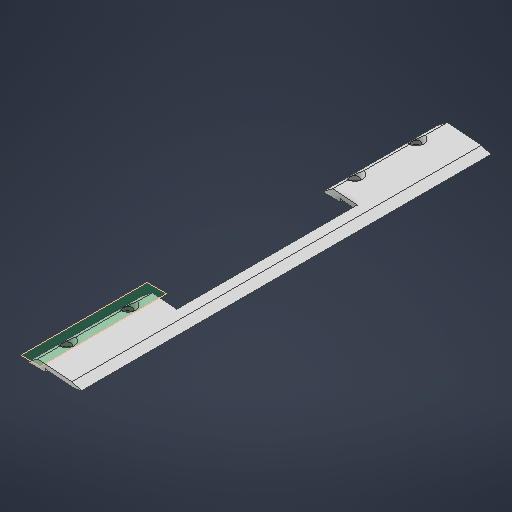
# Autodesk Inventor part: przódv3
Saved by Autodesk Inventor 2026.2 (Build 302298010, 298A)
## iProperties
Created: 2026-05-13
Part Number: przódv3
Material: Generic
Document SubType Name: Modeling
Designer: karol
Density: 1 g/cm^3
Appearance: Default
Author: karol
Autodesk Inventor part; units mm, degrees
ref_plane "YZ Plane" through (0, 0, 0) normal (1, 0, 0) x (0, 1, 0)
ref_plane "XZ Plane" through (0, 0, 0) normal (0, 1, 0) x (-1, 0, 0)
ref_plane "XY Plane" through (0, 0, 0) normal (0, 0, 1) x (1, 0, 0)
sketch "Sketch1" plane through (0, 0, 0) normal (0, 0, 1) x (1, 0, 0)
  line L0 (0.1259, -2.059) -> (22.8182, -5.8085) projected
  line L1 (22.8182, -5.8085) -> (24.1224, 2.0845) projected
  line L2 (11.2963, 4.2038) -> (24.1224, 2.0845) projected
  line L3 (11.2963, 4.2038) -> (0.6373, 1.036) projected
  line L4 (0.6373, 1.036) -> (0.1259, -2.059) projected
  line L5 (0, 0) -> (0, 2) projected
  line L6 (0, 2) -> (-6.5, 2) projected
  line L7 (-6.5, 0) -> (-6.5, 2) projected
  line L8 (0, 0) -> (-6.5, 0) projected
  line L9 (-6.5, 2) -> (0, 2)
  line L10 (-6.5, 2) -> (0, 2)
  line L11 (0, 2) -> (0, 3.5)
  line L12 (0, 3.5) -> (11.2963, 4.2038)
  line L13 (-2.7633, 4.8337) -> (11.2028, 5.7038)
  line L14 (11.2028, 5.7038) -> (11.2963, 4.2038)
  line L15 (-2.7633, 4.8337) -> (-6.5, 2)
  dimension "d0" = 1.5
  dimension "d1" = 1.5
  dimension "d2" = 4.6896
  constraints: 14 end point, 3 perpendicular, 1 horizontal, 1 parallel
  measures "d0" distance of L5.end L11.end
  measures "d1" vertical distance of L13.end L2.start
  measures "d2" distance of L13.start L6.end
extrude "Extrusion1" add sketch "Sketch1" against normal blind 50 contours L12 L11 L6 L15 L13 L14
sketch "Sketch2" plane through (0, 0, -50) normal (0, 0, -1) x (-1, 0, 0)
  line L0 (2.7633, 4.8337) -> (-11.2028, 5.7038) projected
  line L1 (-11.2028, 5.7038) -> (-5.2144, 5.3307)
  line L2 (-11.2028, 5.7038) -> (-11.2963, 4.2038) projected
  line L3 (-11.2028, 5.7038) -> (-11.2963, 4.2038)
  line L4 (-11.2963, 4.2038) -> (-5.3079, 3.8307)
  line L5 (-5.3079, 3.8307) -> (-5.2144, 5.3307)
  point P0 (0, 0)
  dimension "d5" = 6
  dimension "d6" = 6
  constraints: 8 end point, 1 collinear, 1 perpendicular, 1 point on line
  measures "d5" distance of L0.end L1.end
  measures "d6" distance of L2.end L4.end
extrude "Extrusion2" add sketch "Sketch2" along normal blind 50
sketch "Sketch3" plane through (0, 0, -100) normal (0, 0, -1) x (-1, 0, 0)
  line L0 (-5.3079, 3.8307) -> (-5.2144, 5.3307) projected
  line L1 (-5.2144, 5.3307) -> (-11.2028, 5.7038) projected
  line L2 (-11.2028, 5.7038) -> (-11.2963, 4.2038) projected
  line L3 (-11.2963, 4.2038) -> (-5.3079, 3.8307) projected
  line L4 (-5.2144, 5.3307) -> (-5.3079, 3.8307) projected
  line L5 (-5.3079, 3.8307) -> (0, 3.5) projected
  line L6 (0, 3.5) -> (0, 2) projected
  line L7 (0, 2) -> (6.5, 2) projected
  line L8 (6.5, 2) -> (2.7633, 4.8337) projected
  line L9 (2.7633, 4.8337) -> (-5.2144, 5.3307) projected
  point P0 (0, 0)
extrude "Extrusion3" add sketch "Sketch3" along normal blind 50
sketch "Sketch4" plane through (0, 0, 0) normal (0, 0, 1) x (1, 0, 0)
  line L0 (0.1259, -2.059) -> (22.8182, -5.8085) projected
  line L1 (22.8182, -5.8085) -> (24.1224, 2.0845) projected
  line L2 (11.2963, 4.2038) -> (24.1224, 2.0845) projected
  line L3 (11.2963, 4.2038) -> (0.6373, 1.036) projected
  line L4 (0.6373, 1.036) -> (0.1259, -2.059) projected
  line L5 (15.9878, 3.4286) -> (5.1621, 5.3274)
  line L6 (-2.7633, 4.8337) -> (11.2028, 5.7038) projected
  line L7 (-6.5, 2) -> (0, 2) projected
  line L8 (0, 2) -> (0, 3.5) projected
  line L9 (0, 3.5) -> (11.2963, 4.2038) projected
  line L10 (11.2963, 4.2038) -> (11.2028, 5.7038) projected
  line L11 (11.2028, 5.7038) -> (-2.7633, 4.8337) projected
  line L12 (-2.7633, 4.8337) -> (-6.5, 2) projected
  point P0 (0, 0)
  point P1 (11.2933, 4.252)
  constraints: 2 end point, 2 point on line
extrude "Extrusion4" cut sketch "Sketch4" against normal blind 150 contours L5 L6 L10
sketch "Sketch5" plane through (0, 0, 0) normal (0, 0, 1) x (1, 0, 0)
  line L0 (11.2933, 4.252) -> (5.1621, 5.3274) projected
  line L1 (5.1621, 5.3274) -> (-2.7633, 4.8337) projected
  line L2 (-2.7633, 4.8337) -> (-6.5, 2) projected
  line L3 (-6.5, 2) -> (0, 2) projected
  line L4 (0, 2) -> (0, 3.5) projected
  line L5 (0, 3.5) -> (11.2963, 4.2038) projected
  line L6 (11.2963, 4.2038) -> (11.2933, 4.252) projected
  line L7 (11.2963, 4.2038) -> (5.1621, 5.3274)
  line L8 (5.1621, 5.3274) -> (4.8831, 3.8042)
  line L9 (4.8831, 3.8042) -> (8.2292, 3.1913)
  line L10 (8.2292, 3.1913) -> (11.2963, 4.2038)
  line L11 (8.2292, 3.1913) -> (11.2963, 4.2038)
  point P0 (0, 0)
  constraints: 10 end point, 2 perpendicular, 1 collinear, 1 point on line
extrude "Extrusion5" add sketch "Sketch5" against normal blind 50 contours L10 L9 L5
sketch "Sketch6" plane through (0, 0, -150) normal (0, 0, -1) x (-1, 0, 0)
  line L0 (-5.1621, 5.3274) -> (-5.2152, 5.3181) projected
  line L1 (-5.2152, 5.3181) -> (-5.3079, 3.8307) projected
  line L2 (-11.2963, 4.2038) -> (-5.3079, 3.8307) projected
  line L3 (-11.2963, 4.2038) -> (-8.2292, 3.1913) projected
  line L4 (-8.2292, 3.1913) -> (-4.8831, 3.8042) projected
  line L5 (-4.8831, 3.8042) -> (0, 3.5) projected
  line L6 (0, 3.5) -> (0, 2) projected
  line L7 (0, 2) -> (6.5, 2) projected
  line L8 (6.5, 2) -> (2.7633, 4.8337) projected
  line L9 (2.7633, 4.8337) -> (-5.1621, 5.3274) projected
  line L10 (-8.2292, 3.1913) -> (-4.8831, 3.8042)
  line L11 (-11.2963, 4.2038) -> (-8.2292, 3.1913)
  point P0 (0, 0)
  constraints: 4 end point, 2 collinear
extrude "Extrusion6" add sketch "Sketch6" against normal blind 50
sketch "Sketch8" plane through (0, 0, 0) normal (0, 0, 1) x (1, 0, 0)
  line L0 (0, 3.5) -> (0, 2) projected
  line L1 (0, 3.0019) -> (6.912, 3.4326)
  line L2 (8.2292, 3.1913) -> (4.8831, 3.8042) projected
  line L3 (5.1621, 5.3274) -> (-2.7633, 4.8337) projected
  line L4 (11.2933, 4.252) -> (5.1621, 5.3274) projected
  line L5 (5.1621, 5.3274) -> (-2.7633, 4.8337) projected
  line L6 (-2.7633, 4.8337) -> (-6.5, 2) projected
  line L7 (-6.5, 2) -> (0, 2) projected
  line L8 (0, 2) -> (0, 3.5) projected
  line L9 (0, 3.5) -> (4.8831, 3.8042) projected
  line L10 (4.8831, 3.8042) -> (8.2292, 3.1913) projected
  line L11 (8.2292, 3.1913) -> (11.2963, 4.2038) projected
  line L12 (11.2963, 4.2038) -> (11.2933, 4.252) projected
  point P0 (0, 0)
  dimension "d19" = 2
  constraints: 2 end point, 2 point on line, 1 parallel
  measures "d19" distance between parallel lines of L3 L1
extrude "Extrusion8" add sketch "Sketch8" against normal blind 50 contours L9 L2 L1 L0
sketch "Sketch9" plane through (0, 0, -150) normal (0, 0, -1) x (-1, 0, 0)
  line L0 (-4.8831, 3.8042) -> (0, 3.5) projected
  line L1 (-5.1621, 5.3274) -> (-5.2152, 5.3181) projected
  line L2 (-5.2152, 5.3181) -> (-5.3079, 3.8307) projected
  line L3 (-11.2963, 4.2038) -> (-5.3079, 3.8307) projected
  line L4 (-11.2963, 4.2038) -> (-8.2292, 3.1913) projected
  line L5 (-8.2292, 3.1913) -> (-6.912, 3.4326) projected
  line L6 (-6.912, 3.4326) -> (0, 3.0019) projected
  line L7 (0, 3.0019) -> (0, 2) projected
  line L8 (0, 2) -> (6.5, 2) projected
  line L9 (6.5, 2) -> (2.7633, 4.8337) projected
  line L10 (2.7633, 4.8337) -> (-5.1621, 5.3274) projected
  line L11 (-6.912, 3.4326) -> (-4.8831, 3.8042)
  line L12 (0, 3.0019) -> (0, 3.5)
  point P0 (0, 0)
  constraints: 4 end point, 1 vertical
extrude "Extrusion9" add sketch "Sketch9" against normal blind 50 contours L0 L12 L6 L11
sketch "Sketch10" plane through (0, 0, -150) normal (0, 0, -1) x (-1, 0, 0)
  line L0 (-5.3079, 3.8307) -> (-11.2963, 4.2038) projected
  line L1 (-6.912, 3.4326) -> (-8.2292, 3.1913) projected
  line L2 (-11.2963, 4.2038) -> (-8.2292, 3.1913)
  line L3 (-8.2292, 3.1913) -> (-8.0187, 3.2298)
  line L4 (-8.0187, 3.2298) -> (-11.2963, 4.2038)
  point P0 (0, 0)
  dimension "d24" = 0.214
  constraints: 6 end point, 1 point on line
  measures "d24" distance of L1.end L3.end
extrude "Extrusion10" cut sketch "Sketch10" against normal blind 150
sketch "Szkic11" plane through (0, 0, -100) normal (0, 0, 1) x (1, 0, 0)
  line L0 (8.0187, 3.2298) -> (11.2963, 4.2038) projected
  line L1 (5.3079, 3.8307) -> (11.2963, 4.2038) projected
  line L2 (5.3079, 3.8307) -> (5.2152, 5.3181) projected
  line L3 (5.2152, 5.3181) -> (5.1621, 5.3274) projected
  line L4 (-2.7633, 4.8337) -> (5.1621, 5.3274) projected
  line L5 (-6.5, 2) -> (-2.7633, 4.8337) projected
  line L6 (0, 2) -> (-6.5, 2) projected
  line L7 (0, 3.0019) -> (0, 2) projected
  line L8 (0, 3.0019) -> (6.912, 3.4326) projected
  line L9 (6.912, 3.4326) -> (8.0187, 3.2298) projected
  line L10 (5.2152, 5.3181) -> (5.3388, 3.3346)
  point P0 (0, 0)
  constraints: 2 end point, 2 point on line
extrude "Wyciągnięcie proste11" cut sketch "Szkic11" against normal blind 8 contours L10 L8 L7 L6 L5 L4 L3 L2
sketch "Szkic12" plane through (0, 0, -50) normal (0, 0, -1) x (-1, 0, 0)
  line L0 (-11.2963, 4.2038) -> (-8.0187, 3.2298) projected
  line L1 (-8.0187, 3.2298) -> (-6.912, 3.4326) projected
  line L2 (-6.912, 3.4326) -> (0, 3.0019) projected
  line L3 (0, 3.0019) -> (0, 2) projected
  line L4 (0, 2) -> (6.5, 2) projected
  line L5 (6.5, 2) -> (2.7633, 4.8337) projected
  line L6 (2.7633, 4.8337) -> (-5.1621, 5.3274) projected
  line L7 (-5.1621, 5.3274) -> (-11.2933, 4.252) projected
  line L8 (-11.2933, 4.252) -> (-11.2963, 4.2038) projected
  line L9 (-5.2152, 5.3181) -> (-5.3079, 3.8307) projected
  line L10 (-5.2152, 5.3181) -> (-5.3388, 3.3346)
  point P0 (0, 0)
  constraints: 2 end point, 1 perpendicular, 1 point on line
extrude "Wyciągnięcie proste12" cut sketch "Szkic12" against normal blind 8 contours L7 L6 L5 L4 L3 L2 L10 L9
sketch "Szkic13" plane through (-6.5, 2, 0) normal (0, -1, 0) x (1, 0, 0)
  circle A0 centre (3.25, -11) radius 1.55
  circle A1 centre (3.25, -33.5) radius 1.55
  circle A2 centre (3.25, -116.5) radius 1.55
  circle A3 centre (3.25, -139) radius 1.55
  line L0 (6.5, -150) -> (0, -150) projected
  line L1 (0, 0) -> (6.5, 0) projected
  line L2 (0, -108) -> (0, -150) projected
  line L3 (0, 0) -> (0, -42) projected
  dimension "d31" = 3.1
  dimension "d32" = 3.1
  dimension "d33" = 3.1
  dimension "d34" = 3.1
  dimension "d35" = 11
  dimension "d36" = 33.5
  dimension "d37" = 33.5
  dimension "d38" = 11
  dimension "d39" = 3.25
  dimension "d40" = 3.25
  dimension "d41" = 3.25
  dimension "d42" = 3.25
  constraints: 4 centre point
  measures "d31" diameter of A0
  measures "d32" diameter of A1
  measures "d33" diameter of A2
  measures "d34" diameter of A3
  measures "d35" distance from line of L0 A3.centre
  measures "d36" distance from line of L0 A2.centre
  measures "d37" distance from line of L1 A1.centre
  measures "d38" distance from line of L1 A0.centre
  measures "d39" distance from line of L2 A3.centre
  measures "d40" distance from line of L2 A2.centre
  measures "d41" distance from line of L3 A1.centre
  measures "d42" distance from line of L3 A0.centre
extrude "Wyciągnięcie proste13" cut sketch "Szkic13" against normal blind 3
ref_plane "Płaszczyzna konstrukcyjna1" through (-6.5, 5, 0) normal (0, -1, 0) x (1, 0, 0)
sketch "Szkic15" plane through (-6.5, 5, 0) normal (0, -1, 0) x (1, 0, 0)
  arc A0 (3.7367, -9.5284) -> (3.7367, -12.4716) centre (3.25, -11) ccw projected
  arc A1 (3.7367, -32.0284) -> (3.7367, -34.9716) centre (3.25, -33.5) ccw projected
  arc A2 (3.7367, -115.0284) -> (3.7367, -117.9716) centre (3.25, -116.5) ccw projected
  arc A3 (3.7367, -137.5284) -> (3.7367, -140.4716) centre (3.25, -139) ccw projected
  point P0 (6.5, 0)
hole "Otwór2" at (-3.25, 5, -11) at (-3.25, 5, -33.5) at (-3.25, 5, -139) at (-3.25, 5, -116.5) direction (0, -1, 0) diameter 3.1 depth 3 tip angle 118 countersink diameter 6.3 countersink angle 90
sketch "Szkic16" plane through (0, 0, 0) normal (0, 0, 1) x (1, 0, 0)
  line L0 (6.912, 3.4326) -> (0, 3.0019) projected
  line L1 (11.2963, 4.2038) -> (8.0187, 3.2298) projected
  line L2 (6.912, 3.4326) -> (8.0187, 3.2298)
  line L3 (8.0187, 3.2298) -> (6.912, 3.4326)
  line L4 (13.2517, 2.7421) -> (2.4584, 0.0677) projected
  line L5 (6.912, 3.4326) -> (10.8977, 2.1588)
  line L6 (-2.7633, 4.8337) -> (5.1621, 5.3274) projected
  line L7 (5.1621, 5.3274) -> (13.2517, 2.7421)
  line L8 (5.1621, 5.3274) -> (11.2933, 4.252) projected
  line L9 (5.1621, 5.3274) -> (11.2933, 4.252)
  line L10 (11.2933, 4.252) -> (11.2963, 4.2038)
  line L11 (11.2963, 4.2038) -> (9.9395, 3.8006)
  line L12 (8.0187, 3.2298) -> (9.9395, 3.8006)
  line L13 (13.2517, 2.7421) -> (10.8977, 2.1588)
  point P0 (0, 0)
  constraints: 18 end point, 4 collinear, 4 point on line, 1 parallel
extrude "Wyciągnięcie proste14" add sketch "Szkic16" against normal blind 150 contours L7 L4 L5 L2 L1
sketch "Szkic17" plane through (0, 0, 0) normal (0, 0, 1) x (1, 0, 0)
  line L0 (-2.7633, 4.8337) -> (5.1621, 5.3274) projected
  line L1 (13.2517, 2.7421) -> (9.9395, 3.8006) projected
  line L2 (5.1621, 5.3274) -> (9.9395, 3.8006)
  line L3 (9.9395, 3.8006) -> (11.2963, 4.2038) projected
  line L4 (9.9395, 3.8006) -> (11.2963, 4.2038)
  line L5 (11.2963, 4.2038) -> (11.2933, 4.252) projected
  line L6 (11.2963, 4.2038) -> (11.2933, 4.252)
  line L7 (11.2933, 4.252) -> (5.1621, 5.3274) projected
  line L8 (11.2933, 4.252) -> (5.1621, 5.3274)
  point P0 (0, 0)
  constraints: 8 end point, 4 collinear
extrude "Wyciągnięcie proste15" cut sketch "Szkic17" against normal blind 150
sketch "Szkic18" plane through (0, 0, 0) normal (0, 0, 1) x (1, 0, 0)
  line L0 (6.912, 3.4326) -> (10.8977, 2.1588) projected
  line L1 (10.8977, 2.1588) -> (6.912, 3.4326)
  line L2 (10.8977, 2.1588) -> (13.2517, 2.7421) projected
  line L3 (6.912, 3.4326) -> (10.8977, 2.1588)
  line L4 (13.2517, 2.7421) -> (5.1621, 5.3274) projected
  line L5 (13.2517, 2.7421) -> (5.1621, 5.3274)
  line L6 (5.1621, 5.3274) -> (2.2957, 5.1488)
  line L7 (5.1621, 5.3274) -> (-2.7633, 4.8337) projected
  line L8 (10.8977, 2.1588) -> (1.6648, 5.1095)
  point P0 (0, 0)
  point P1 (1.6648, 5.1095)
  constraints: 10 end point, 3 collinear, 2 point on line, 1 parallel
extrude "Wyciągnięcie proste16" add sketch "Szkic18" against normal blind 150
sketch "Szkic19" plane through (0, 0, 0) normal (0, 0, 1) x (1, 0, 0)
  line L0 (5.1621, 5.3274) -> (-2.7633, 4.8337) projected
  line L1 (-2.7633, 4.8337) -> (-6.5, 2) projected
  line L2 (-6.5, 2) -> (0, 2) projected
  line L3 (0, 2) -> (0, 3.0019) projected
  line L4 (0, 3.0019) -> (6.912, 3.4326) projected
  line L5 (6.912, 3.4326) -> (10.8977, 2.1588) projected
  line L6 (10.8977, 2.1588) -> (13.2517, 2.7421) projected
  line L7 (13.2517, 2.7421) -> (5.1621, 5.3274) projected
  line L8 (0, 3.0019) -> (10.8977, 2.1588)
  line L9 (-2.7633, 4.8337) -> (5.1621, 5.3274)
  line L10 (5.1621, 5.3274) -> (13.2517, 2.7421) projected
  line L11 (0, 3.0019) -> (6.912, 3.4326) projected
  point P0 (0, 0)
  constraints: 4 end point, 1 parallel, 1 point on line
extrude "Wyciągnięcie proste17" add sketch "Szkic19" against normal blind 150 contours L8 L4 L5
sketch "Szkic20" plane through (0, 0, 0) normal (0, 0, 1) x (1, 0, 0)
  line L0 (-2.7633, 4.8337) -> (5.1621, 5.3274) projected
  line L1 (-2.7633, 4.8337) -> (9.7322, 3.8669)
  line L2 (5.1621, 5.3274) -> (13.2517, 2.7421) projected
  line L3 (0, 3.0019) -> (10.8977, 2.1588) projected
  point P0 (0, 0)
  constraints: 2 end point, 1 parallel, 1 point on line
extrude "Wyciągnięcie proste18" cut sketch "Szkic20" against normal blind 150
sketch "Szkic21" plane through (0, 3.0019, -42) normal (-0.0621796, 0.998065, 0) x (0.998065, 0.0621796, 0)
  line L0 (5.3492, 66) -> (0, 66) projected
  line L1 (0, 0) -> (0, 66) projected
  line L2 (0, 0) -> (5.3492, 0) projected
  line L3 (5.3492, 0) -> (5.3492, 8) projected
  line L4 (6.9254, 8) -> (5.3492, 8) projected
  line L5 (6.9254, 58) -> (6.9254, 8) projected
  line L6 (5.3492, 58) -> (6.9254, 58) projected
  line L7 (5.3492, 58) -> (5.3492, 66) projected
  line L8 (0, 66) -> (-0.0623, 66) projected
  line L9 (-0.0623, 66) -> (5.3492, 66)
  line L10 (5.3492, 66) -> (5.3492, 0)
  line L11 (5.3492, 0) -> (-0.0623, 0)
  line L12 (-0.0623, 0) -> (-0.0623, 66)
  point P0 (-0.1867, -42)
  constraints: 8 end point, 2 parallel, 1 horizontal, 1 perpendicular
extrude "Wyciągnięcie proste19" cut sketch "Szkic21" against normal blind 150 contours L7 L10 L3 L2 L1 L0 | L1 L11 L12 L8
sketch "Szkic22" plane through (9.7322, 3.8669, 0) normal (0.0771416, 0.9970201, 0) x (0.9970201, -0.0771416, 0)
  line L0 (-5.5305, 42) -> (-5.5305, 108) projected
  line L1 (-5.5305, 108) -> (-3.5305, 108)
  line L2 (-3.5305, 108) -> (-3.5305, 42)
  line L3 (-3.5305, 42) -> (-5.5305, 42)
  line L4 (-5.5305, 42) -> (-5.5305, 108)
  point P0 (-9.4049, 0)
  dimension "d72" = 2
  constraints: 8 end point, 2 parallel, 1 horizontal, 1 perpendicular
  measures "d72" distance of L2.end L3.end
extrude "Wyciągnięcie proste20" cut sketch "Szkic22" against normal blind 150
body "Solid1"
